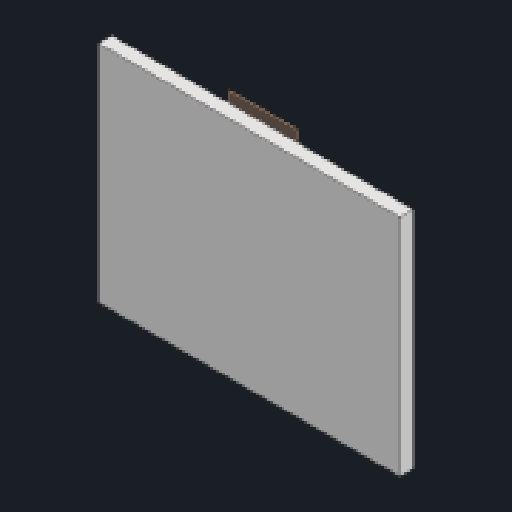
# Autodesk Inventor part: front_metal_gear_holder
Saved by Autodesk Inventor 2023 (Build 270158000, 158)
## iProperties
Created: 2024-04-25
Part Number: front_metal_gear_holder
Material: Generic
Document SubType Name: Modeling
Designer: szymo
Density: 1 g/cm^3
Appearance: Default
Author: szymo
Autodesk Inventor part; units mm, degrees
ref_plane "YZ Plane" through (0, 0, 0) normal (1, 0, 0) x (0, 1, 0)
ref_plane "XZ Plane" through (0, 0, 0) normal (0, 1, 0) x (-1, 0, 0)
ref_plane "XY Plane" through (0, 0, 0) normal (0, 0, 1) x (1, 0, 0)
ref_plane "Work Plane1" through (0, 0, 0) normal (0, 0, 1) x (1, 0, 0)
sketch "Sketch1" plane through (0, 0, 0) normal (0, 0, 1) x (1, 0, 0)
  line L0 (-12, 33.5) -> (-18, 33.5) projected
  line L1 (-18, 0) -> (-18, 33.5) projected
  line L2 (-18, 0) -> (-12, 0) projected
  line L3 (-12, 0) -> (-12, 33.5) projected
  line L4 (27, 33.5) -> (21, 33.5) projected
  line L5 (21, 0) -> (21, 33.5) projected
  line L6 (21, 0) -> (27, 0) projected
  line L7 (27, 0) -> (27, 33.5) projected
  line L8 (-18, 33.5) -> (27, 33.5)
  line L9 (27, 33.5) -> (27, 0)
  line L10 (27, 0) -> (-18, 0)
  line L11 (-18, 0) -> (-18, 33.5)
  point P0 (0, 0)
  constraints: 8 end point, 2 parallel, 1 horizontal, 1 perpendicular
ref_plane "Work Plane2" through (-69.2, 0, 2) normal (0, 0, -1) x (0, 1, 0)
extrude "Extrusion1" add sketch "Sketch1" along normal up to surface (2 mm away)
body "Solid1"
